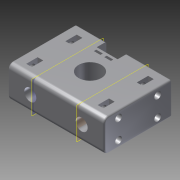
# Autodesk Inventor part: V5 Z Bottom Center
Saved by Autodesk Inventor 2012 (Build 160160000, 160)
## iProperties
Created: 2013-01-29
Part Number: V5 Z Bottom Center
Material: Default
Document SubType Name: Modeling
Designer: mce
Density: 1 g/cm^3
Author: mce
Autodesk Inventor part; units mm, degrees
ref_plane "YZ Plane" through (0, 0, 0) normal (1, 0, 0) x (0, 1, 0)
ref_plane "XZ Plane" through (0, 0, 0) normal (0, 1, 0) x (-1, 0, 0)
ref_plane "XY Plane" through (0, 0, 0) normal (0, 0, 1) x (1, 0, 0)
sketch "Sketch1" plane through (0, 0, 0) normal (0, 0, 1) x (1, 0, 0)
  line L0 (0, 0) -> (60, 0)
  line L1 (60, 0) -> (60, 42.4)
  line L2 (60, 42.4) -> (0, 42.4)
  line L3 (0, 42.4) -> (0, 0)
  circle A0 centre (30, 21.2) radius 5
  dimension "d0" = 42.4
  dimension "d1" = 60
  dimension "d2" = 21.2
  dimension "d3" = 30
  dimension "d4" = 10
  constraints: 8 end point, 2 horizontal, 2 vertical, 1 centre point
  measures "d0" distance of L2.end L0.start
  measures "d1" distance of L0.start L0.end
  measures "d2" distance from line of L2 A0.centre
  measures "d3" distance from line of L3 A0.centre
  measures "d4" diameter of A0
extrude "Extrusion1" add sketch "Sketch1" along normal blind 20
sketch "Sketch2" plane through (0, 0, 0) normal (-1, 0, 0) x (0, 0, 1)
  line L0 (20, 0) -> (20, 42.4) projected
  line L1 (0, 42.4) -> (20, 42.4) projected
  line L2 (0, 42.4) -> (0, 0) projected
  line L3 (0, 0) -> (20, 0) projected
  circle A0 centre (4, 33.4) radius 2.1
  circle A1 centre (16, 33.4) radius 2.1
  circle A2 centre (4, 9) radius 2.1
  circle A3 centre (16, 9) radius 2.1
  dimension "d7" = 4.2
  dimension "d8" = 4
  dimension "d9" = 9
  dimension "d10" = 9
  dimension "d11" = 4
  dimension "d12" = 4
  dimension "d13" = 4
  dimension "d14" = 9
  dimension "d15" = 9
  constraints: 4 centre point, 3 equal radius
  measures "d7" diameter of A0
  measures "d8" distance from line of L2 A0.centre
  measures "d9" distance from line of L1 A0.centre
  measures "d10" distance from line of L1 A1.centre
  measures "d11" distance from line of L0 A1.centre
  measures "d12" distance from line of L0 A3.centre
  measures "d13" distance from line of L2 A2.centre
  measures "d14" distance from line of L3 A2.centre
  measures "d15" distance from line of L3 A3.centre
extrude "Extrusion2" cut sketch "Sketch2" against normal up to next contours A0 | A1 | A2 | A3
fillet "Fillet1" radius 1 10 edges at (0, 42.4, 10) (30, 42.4, 20) (30, 42.4, 0) (60, 42.4, 10) (0, 21.2, 20) (0, 21.2, 0) (60, 21.2, 20) (60, 21.2, 0) (0, 0, 10) (60, 0, 10)
fillet "Fillet2" radius 3 6 edges at (30, 0, 20) (0.2929, 0.2929, 19.7071) (59.7071, 0.2929, 19.7071) (59.7071, 0.2929, 0.2929) (0.2929, 0.2929, 0.2929) (30, 0, 0)
sketch "Sketch3" plane through (0, 0, 20) normal (0, 0, 1) x (1, 0, 0)
  line L0 (9.5, 36.95) -> (6, 36.95)
  line L1 (6, 36.95) -> (6, 29.85)
  line L2 (6, 29.85) -> (9.5, 29.85)
  line L3 (9.5, 29.85) -> (9.5, 36.95)
  line L4 (9.5, 12.55) -> (6, 12.55)
  line L5 (6, 12.55) -> (6, 5.45)
  line L6 (6, 5.45) -> (9.5, 5.45)
  line L7 (9.5, 5.45) -> (9.5, 12.55)
  line L8 (54, 36.95) -> (50.5, 36.95)
  line L9 (50.5, 36.95) -> (50.5, 29.85)
  line L10 (50.5, 29.85) -> (54, 29.85)
  line L11 (54, 29.85) -> (54, 36.95)
  line L12 (54, 12.55) -> (50.5, 12.55)
  line L13 (50.5, 12.55) -> (50.5, 5.45)
  line L14 (50.5, 5.45) -> (54, 5.45)
  line L15 (54, 5.45) -> (54, 12.55)
  line L16 (0, 41.4) -> (0, 3) projected
  line L17 (60, 3) -> (60, 41.4) projected
  line L18 (59, 42.4) -> (1, 42.4) projected
  line L19 (1, 0) -> (59, 0) projected
  point P0 (0, 0)
  point P1 (50.5, 9)
  dimension "d20" = 3.5
  dimension "d21" = 7.1
  dimension "d22" = 6
  dimension "d23" = 6
  dimension "d24" = 5.45
  dimension "d25" = 5.45
  constraints: 32 end point, 8 collinear, 4 equal length, 3 horizontal, 3 vertical, 1 midpoint
  measures "d20" distance of L0.start L0.end
  measures "d21" distance of L0.end L1.end
  measures "d22" distance between parallel lines of L16 L1
  measures "d23" distance between parallel lines of L17 L11
  measures "d24" distance between parallel lines of L0 L18
  measures "d25" distance between parallel lines of L6 L19
extrude "Extrusion3" cut sketch "Sketch3" against normal blind 20
ref_plane "Work Plane2" through (44, 41.4, 19) normal (1, 0, 0) x (0, 0, -1)
ref_plane "Work Plane3" through (16, 41.4, 1) normal (-1, 0, 0) x (0, 0, 1)
sketch "Sketch8" plane through (44, 41.4, 19) normal (1, 0, 0) x (0, 0, -1)
  circle A0 centre (3, -8) radius 2.1
  circle A1 centre (15, -8) radius 2.1
  circle A2 centre (15, -32.4) radius 2.1
  circle A3 centre (3, -32.4) radius 2.1
  circle A4 centre (3, -32.4) radius 2.1 projected
  circle A5 centre (15, -32.4) radius 2.1 projected
  circle A6 centre (15, -8) radius 2.1 projected
  circle A7 centre (3, -8) radius 2.1 projected
  point P0 (19, -41.4)
  constraints: 8 concentric, 4 centre point
extrude "Extrusion9" add sketch "Sketch8" against normal up to surface (28 mm away)
sketch "Sketch11" plane through (1, 0, 3) normal (0, -1, 0) x (1, 0, 0)
  circle A0 centre (13, 7) radius 2.05
  circle A1 centre (45, 7) radius 2.05
  line L0 (58, 17) -> (0, 17) projected
  line L1 (-1, 14) -> (-1, 0) projected
  line L2 (59, 0) -> (59, 14) projected
  point P0 (-1, -3)
  dimension "d61" = 10
  dimension "d62" = 10
  dimension "d63" = 4.1
  dimension "d64" = 14
  dimension "d65" = 14
  constraints: 2 centre point, 1 equal radius
  measures "d61" distance from line of A0.centre L0
  measures "d62" distance from line of L0 A1.centre
  measures "d63" diameter of A0
  measures "d64" distance from line of L1 A0.centre
  measures "d65" distance from line of L2 A1.centre
extrude "Extrusion11" cut sketch "Sketch11" against normal up to next
sketch "Sketch12" plane through (1, 0, 3) normal (0, -1, 0) x (1, 0, 0)
  circle A0 centre (45, 7) radius 2.05 projected
  circle A1 centre (13, 7) radius 2.05 projected
  circle A2 centre (13, 7) radius 3.75
  circle A3 centre (45, 7) radius 3.75
  point P0 (-1, -3)
  dimension "d68" = 7.5
  constraints: 2 centre point, 2 coincident, 1 equal radius
  measures "d68" diameter of A2
extrude "Extrusion12" cut sketch "Sketch12" against normal blind 6
sketch "Sketch14" plane through (1, 42.4, 1) normal (0, 1, 0) x (1, 0, 0)
  line L0 (18, -19) -> (31, -19)
  line L1 (31, -19) -> (31, -9)
  line L2 (31, -9) -> (18, -9)
  line L3 (18, -9) -> (18, -19)
  line L4 (0, -19) -> (58, -19) projected
  line L5 (59, -18) -> (59, 0) projected
  line L6 (-1, 0) -> (-1, -18) projected
  point P0 (-1, 1)
  dimension "d71" = 13
  dimension "d72" = 10
  dimension "d90" = 19
  constraints: 8 end point, 2 vertical, 1 collinear, 1 horizontal
  measures "d71" distance of L0.start L0.end
  measures "d72" distance of L2.end L0.start
  measures "d90" distance between parallel lines of L6 L3
extrude "Extrusion13" cut sketch "Sketch14" against normal blind 6
sketch "Sketch15" plane through (1, 42.4, 1) normal (0, 1, 0) x (1, 0, 0)
  circle A0 centre (21.25, -14) radius 1.05
  circle A1 centre (27.75, -14) radius 1.05
  line L0 (31, -19) -> (18, -19) projected
  line L1 (18, -9) -> (18, -19) projected
  point P0 (-1, 1)
  point P1 (15, -9.45)
  dimension "d76" = 2.1
  dimension "d77" = 5
  dimension "d78" = 5
  dimension "d79" = 6.5
  dimension "d80" = 3.25
  constraints: 2 centre point, 1 equal radius, 1 other
  measures "d76" diameter of A0
  measures "d77" distance from line of A0.centre L0
  measures "d78" distance from line of L0 A1.centre
  measures "d79" distance of A1.centre A0.centre
extrude "Extrusion14" cut sketch "Sketch15" against normal blind 14
sketch "Sketch16" plane through (0, 0, 20) normal (0, 0, 1) x (1, 0, 0)
  line L0 (32, 36.4) -> (19, 36.4) projected
  line L1 (20.2, 34.9) -> (24.3, 34.9)
  line L2 (24.3, 34.9) -> (24.3, 33.4)
  line L3 (24.3, 33.4) -> (20.2, 33.4)
  line L4 (20.2, 33.4) -> (20.2, 34.9)
  line L5 (26.7, 34.9) -> (30.8, 34.9)
  line L6 (30.8, 34.9) -> (30.8, 33.4)
  line L7 (30.8, 33.4) -> (26.7, 33.4)
  line L8 (26.7, 33.4) -> (26.7, 34.9)
  point P0 (0, 0)
  dimension "d83" = 4.1
  dimension "d84" = 6.5
  dimension "d85" = 1.2
  dimension "d86" = 1.5
  dimension "d87" = 1.5
  constraints: 16 end point, 3 collinear, 3 vertical, 2 horizontal
  measures "d83" distance of L1.start L1.end
  measures "d84" distance between parallel lines of L8 L4
  measures "d85" distance from line of L0.end L4
  measures "d86" distance between parallel lines of L1 L3
  measures "d87" distance between parallel lines of L0 L1
extrude "Extrusion15" cut sketch "Sketch16" against normal blind 8
sketch "Sketch17" plane through (0, 0, 20) normal (0, 0, 1) x (1, 0, 0)
  circle A0 centre (30, 21.2) radius 5 projected
  circle A1 centre (30, 21.2) radius 7.1
  point P0 (0, 0)
  dimension "d91" = 14.2
  constraints: 1 centre point, 1 coincident
  measures "d91" diameter of A1
extrude "Extrusion16" cut sketch "Sketch17" against normal blind 15.5
sketch "Sketch5" plane through (0, 0, 20) normal (0, 0, 1) x (1, 0, 0)
  circle A0 centre (30, 21.2) radius 5 projected
  circle A1 centre (19, 29.2) radius 1.55
  circle A2 centre (19, 13.2) radius 1.55
  circle A3 centre (41, 29.2) radius 1.55
  circle A4 centre (41, 13.2) radius 1.55
  line L0 (-8.167, 21.2) -> (65.5689, 21.2) construction
  line L1 (30, 46.4359) -> (30, -3.5067) construction
  circle A5 centre (19, 29.2) radius 3.5
  point P0 (0, 0)
  dimension "d31" = 16
  dimension "d32" = 3.1
  dimension "d33" = 22
  dimension "d51" = 7
  constraints: 5 centre point, 4 end point, 3 equal radius, 3 symmetric about line, 2 point on line, 1 coincident, 1 horizontal, 1 vertical
  measures "d31" distance of A2.centre A1.centre
  measures "d32" diameter of A1
  measures "d33" distance of A1.centre A3.centre
  measures "d51" diameter of A5
sketch "Sketch6" plane through (0, 0, 20) normal (0, 0, 1) x (1, 0, 0)
  circle A0 centre (41, 13.2) radius 1.55 projected
  circle A1 centre (41, 29.2) radius 1.55 projected
  circle A2 centre (19, 13.2) radius 1.55 projected
  circle A3 centre (19, 29.2) radius 1.55 projected
  line L0 (20.6166, 32) -> (22.2332, 29.2)
  line L1 (22.2332, 29.2) -> (20.6166, 26.4)
  line L2 (20.6166, 26.4) -> (17.3834, 26.4)
  line L3 (17.3834, 26.4) -> (15.7668, 29.2)
  line L4 (15.7668, 29.2) -> (17.3834, 32)
  line L5 (17.3834, 32) -> (20.6166, 32)
  line L6 (44.2332, 13.2) -> (42.6166, 10.4)
  line L7 (42.6166, 10.4) -> (39.3834, 10.4)
  line L8 (39.3834, 10.4) -> (37.7668, 13.2)
  line L9 (37.7668, 13.2) -> (39.3834, 16)
  line L10 (39.3834, 16) -> (42.6166, 16)
  line L11 (42.6166, 16) -> (44.2332, 13.2)
  line L12 (22.2332, 13.2) -> (20.6166, 10.4)
  line L13 (20.6166, 10.4) -> (17.3834, 10.4)
  line L14 (17.3834, 10.4) -> (15.7668, 13.2)
  line L15 (15.7668, 13.2) -> (17.3834, 16)
  line L16 (17.3834, 16) -> (20.6166, 16)
  line L17 (20.6166, 16) -> (22.2332, 13.2)
  line L18 (37.7668, 29.2) -> (39.3834, 32)
  line L19 (39.3834, 32) -> (42.6166, 32)
  line L20 (42.6166, 32) -> (44.2332, 29.2)
  line L21 (44.2332, 29.2) -> (42.6166, 26.4)
  line L22 (42.6166, 26.4) -> (39.3834, 26.4)
  line L23 (39.3834, 26.4) -> (37.7668, 29.2)
  line L24 (26.1832, 21.2) -> (24.675, 21.2)
  line L25 (24.675, 21.2) -> (24.675, 19.0159)
  line L26 (24.675, 19.0159) -> (26.1832, 19.0159)
  line L27 (26.1832, 19.0159) -> (26.1832, 21.2)
  point P0 (0, 0)
  dimension "d36" = 5.6
  constraints: 56 end point, 6 coincident, 3 equal length, 2 horizontal, 2 parallel, 52 other
  measures "d36" distance between parallel lines of L12 L15
sketch "Sketch7" plane through (0, 0, 0) normal (0, 0, -1) x (-1, 0, 0)
  circle A0 centre (-41, 13.2) radius 1.55 projected
  circle A1 centre (-41, 29.2) radius 1.55 projected
  circle A2 centre (-19, 13.2) radius 1.55 projected
  circle A3 centre (-19, 29.2) radius 1.55 projected
  circle A4 centre (-30, 21.2) radius 5 projected
  line L0 (-45.25, 32.95) -> (-14.75, 32.95)
  line L1 (-14.75, 32.95) -> (-14.75, 9.45)
  line L2 (-14.75, 9.45) -> (-45.25, 9.45)
  line L3 (-45.25, 9.45) -> (-45.25, 32.95)
  point P0 (0, 0)
  dimension "d39" = 23.5
  dimension "d40" = 30.5
  dimension "d41" = 15.25
  dimension "d42" = 11.75
  constraints: 8 end point
  measures "d39" distance between parallel lines of L0 L2
  measures "d40" distance between parallel lines of L1 L3
  measures "d41" distance from line of L3 A4.centre
  measures "d42" distance from line of L0 A4.centre
equation "\"d2\" = 0.5 * d0"
equation "\"d3\" = 0.5 * d1"
equation "\"d10\" = d9"
equation "\"d11\" = d8"
equation "\"d12\" = d8"
equation "\"d13\" = d8"
equation "\"d14\" = d9"
equation "\"d15\" = d9"
equation "\"d23\" = d22"
equation "\"d25\" = d24"
equation "\"d65\" = d64"
equation "\"d41\" = 0.5 * d40"
equation "\"d42\" = 0.5 * d39"
body "Solid1"
